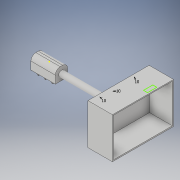
# Autodesk Inventor part: Ampel
Saved by Autodesk Inventor 2019.5 (Build 235369000, 369)
## iProperties
Created: 2021-09-28
Part Number: Ampel
Material: Generisch
Document SubType Name: Modeling
Designer: mritt
Density: 1 g/cm^3
Appearance: Vorgabe
Author: mritt
Autodesk Inventor part; units mm, degrees
ref_plane "YZ Plane" through (0, 0, 0) normal (1, 0, 0) x (0, 1, 0)
ref_plane "XZ Plane" through (0, 0, 0) normal (0, 1, 0) x (-1, 0, 0)
ref_plane "XY Plane" through (0, 0, 0) normal (0, 0, 1) x (1, 0, 0)
sketch "Skizze1" plane through (0, 0, 0) normal (0, 1, 0) x (-1, 0, 0)
  line L0 (34.9666, -12.4012) -> (4.9666, -12.4012)
  line L1 (4.9666, -12.4012) -> (4.9666, -27.4012)
  line L2 (4.9666, -27.4012) -> (34.9666, -27.4012)
  line L3 (34.9666, -27.4012) -> (34.9666, -12.4012)
  circle A0 centre (28.7166, -19.9012) radius 2.5
  circle A1 centre (19.9666, -19.9012) radius 2.5
  circle A2 centre (11.2166, -19.9012) radius 2.5
  line L4 (34.9666, -19.9012) -> (4.9666, -19.9012) construction
  arc A3 (19.9666, -23.4012) -> (19.9666, -16.4012) centre (19.9666, -19.9012) ccw
  arc A4 (28.7166, -23.4012) -> (28.7166, -16.4012) centre (28.7166, -19.9012) ccw
  arc A5 (11.2166, -23.4012) -> (11.2166, -16.4012) centre (11.2166, -19.9012) ccw
  arc A6 (11.2166, -24.4012) -> (11.2166, -15.4012) centre (11.2166, -19.9012) ccw
  arc A7 (19.9666, -24.4012) -> (19.9666, -15.4012) centre (19.9666, -19.9012) ccw
  arc A8 (28.7166, -24.4012) -> (28.7166, -15.4012) centre (28.7166, -19.9012) ccw
  line L5 (11.2166, -16.4012) -> (11.2166, -15.4012)
  line L6 (11.2166, -23.4012) -> (11.2166, -24.4012)
  line L7 (19.9666, -15.4012) -> (19.9666, -16.4012)
  line L8 (19.9666, -23.4012) -> (19.9666, -24.4012)
  line L9 (28.7166, -15.4012) -> (28.7166, -16.4012)
  line L10 (28.7166, -23.4012) -> (28.7166, -24.4012)
  line L11 (33.9666, -26.4012) -> (5.9666, -26.4012)
  line L12 (5.9666, -26.4012) -> (5.9666, -13.4012)
  line L13 (5.9666, -13.4012) -> (33.9666, -13.4012)
  line L14 (33.9666, -13.4012) -> (33.9666, -26.4012)
  point P0 (0, 0)
  dimension "d0" = 30
  dimension "d1" = 5
  dimension "d2" = 5
  dimension "d3" = 5
  dimension "d4" = 15
  dimension "d6" = 0
  dimension "d7" = 0
  dimension "d8" = 0
  dimension "d11" = 6.25
  dimension "d12" = 6.25
  dimension "d14" = 8.75
  dimension "d15" = 3.5
  dimension "d16" = 3.5
  dimension "d17" = 3.5
  dimension "d18" = 4.5
  dimension "d19" = 4.5
  dimension "d20" = 4.5
  dimension "d26" = 1
  dimension "d27" = 1
  dimension "d28" = 1
  dimension "d29" = 1
  constraints: 30 end point, 12 point on circle, 9 centre point, 7 equal length, 6 coincident, 3 perpendicular, 2 horizontal, 2 midpoint, 2 vertical
  measures "d0" distance of L1.end L2.end
  measures "d1" diameter of A0
  measures "d2" diameter of A1
  measures "d3" diameter of A2
  measures "d4" distance of L2.end L0.start
  measures "d6" distance from line of L4 A0.centre
  measures "d7" distance from line of A1.centre L4
  measures "d8" distance from line of A2.centre L4
  measures "d11" distance from line of A2.centre L1
  measures "d12" distance of A0.centre L4.start
  measures "d14" distance of A1.centre A0.centre
  measures "d15" radius of A5
  measures "d16" radius of A3
  measures "d17" radius of A4
  measures "d18" radius of A7
  measures "d19" radius of A6
  measures "d20" radius of A8
  measures "d26" distance between parallel lines of L14 L3
  measures "d27" distance between parallel lines of L0 L13
  measures "d28" distance between parallel lines of L1 L12
  measures "d29" distance between parallel lines of L2 L11
extrude "Extrusion1" add sketch "Skizze1" along normal blind 15 contours L3 L2 L1 L0 | A0 | A1 | A2 | A3 L7 A7 L8 | A4 L9 A8 L10 | A5 L5 A6 L6 | L11 L12 L13 L14
extrude "Extrusion2" add sketch "Skizze1" against normal blind 5 contours A3 L7 A7 L8 | A4 L9 A8 L10 | A5 L5 A6 L6
fillet "Rundung1" radius 6 2 edges at (-19.9666, 15, -12.4012) (-19.9666, 15, -27.4012)
extrude "Extrusion3" add sketch "Skizze1" against normal blind 1 contours L3 L2 L1 L0
extrude "Extrusion4" cut sketch "Skizze1" along normal blind 5 contours A0 | A1 | A2
fillet "Rundung3" radius 0.5 4 edges at (-19.9666, -1, -27.4012) (-4.9666, -1, -19.9012) (-19.9666, -1, -12.4012) (-34.9666, -1, -19.9012)
sketch "Skizze2" plane through (-4.9666, 15, -18.4012) normal (1, 0, 0) x (0, 0, -1)
  circle A0 centre (1.5, -8) radius 3.5
  circle A1 centre (1.5, -8) radius 2.5
  line L0 (-6, -6) -> (-6, -15.5) projected
  line L1 (0, 0) -> (3, 0) projected
  line L2 (-5.5, -16) -> (8.5, -16) projected
  point P0 (-18.4012, -15)
  dimension "d37" = 7
  dimension "d38" = 5
  dimension "d39" = 7.5
  dimension "d41" = 8
  constraints: 2 centre point, 1 coincident
  measures "d37" diameter of A0
  measures "d38" diameter of A1
  measures "d39" distance from line of A0.centre L0
  measures "d41" distance from line of A0.centre L2
extrude "Extrusion5" add sketch "Skizze2" along normal blind 70
sketch "Skizze3" plane through (65.0334, 7, -19.9012) normal (1, 0, 0) x (0, 0, -1)
  line L0 (37.5, 25) -> (-37.5, 25)
  line L1 (-37.5, 25) -> (-37.5, -25)
  line L2 (-37.5, -25) -> (37.5, -25)
  line L3 (37.5, -25) -> (37.5, 25)
  circle A0 centre (0, 0) radius 3.5 projected
  line L4 (37.5, 25) -> (-37.5, -25) construction
  line L5 (-37.5, 25) -> (37.5, -25) construction
  point P0 (-19.9012, -7)
  dimension "d44" = 75
  dimension "d45" = 50
  constraints: 12 end point, 2 midpoint, 2 parallel, 1 horizontal, 1 perpendicular
  measures "d44" distance of L1.end L2.end
  measures "d45" distance of L0.end L1.end
extrude "Extrusion6" add sketch "Skizze3" along normal blind 30
sketch "Skizze4" plane through (65.0334, 7, -19.9012) normal (-1, 0, 0) x (0, 0, 1)
  circle A0 centre (19.9012, 17.6803) radius 5
  circle A1 centre (2.6255, 17.6803) radius 5
  circle A2 centre (-21.2224, 17.6803) radius 5
  point P0 (19.9012, -7)
  dimension "d48" = 10
  dimension "d49" = 10
  dimension "d50" = 10
  constraints: 3 centre point
  measures "d48" diameter of A0
  measures "d49" diameter of A1
  measures "d50" diameter of A2
sketch "Skizze5" plane through (65.0334, 32, 17.5988) normal (0, 1, 0) x (1, 0, 0)
  line L0 (22.9571, 44.9916) -> (27.8876, 44.9916)
  line L1 (27.8876, 44.9916) -> (27.8876, 56.3697)
  line L2 (27.8876, 56.3697) -> (22.9571, 56.3697)
  line L3 (22.9571, 56.3697) -> (22.9571, 44.9916)
  point P0 (-65.0334, 17.5988)
  constraints: 8 end point, 2 parallel, 1 horizontal, 1 perpendicular
sketch "Skizze6" plane through (95.0334, 7, -19.9012) normal (1, 0, 0) x (0, 0, -1)
  line L0 (36, -23.5) -> (-36, -23.5)
  line L1 (-36, -23.5) -> (-36, 23.8)
  line L2 (-36, 23.8) -> (36, 23.8)
  line L3 (36, 23.8) -> (36, -23.5)
  line L4 (-37.5, -25) -> (37.5, -25) projected
  line L5 (-37.5, 25) -> (-37.5, -25) projected
  line L6 (37.5, 25) -> (-37.5, 25) projected
  line L7 (37.5, -25) -> (37.5, 25) projected
  point P0 (-19.9012, -7)
  dimension "d51" = 1.5
  dimension "d52" = 1.5
  dimension "d53" = 1.2
  dimension "d54" = 1.5
  constraints: 8 end point, 2 parallel, 1 horizontal, 1 perpendicular
  measures "d51" distance between parallel lines of L0 L4
  measures "d52" distance between parallel lines of L5 L1
  measures "d53" distance between parallel lines of L2 L6
  measures "d54" distance between parallel lines of L3 L7
extrude "Extrusion7" cut sketch "Skizze6" against normal blind 28 contours L0 L1 L2 L3
